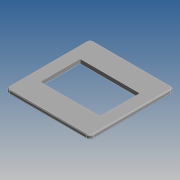
# Autodesk Inventor part: F114DiaReseau
Saved by Autodesk Inventor 2015 SP1 (Build 190203100, 203)
## iProperties
Created: 2017-05-18
Part Number: F114DiaReseau
Material: Générique
Document SubType Name: Modeling
Designer: serge.amoos
Density: 1 g/cm^3
Appearance: Par défaut
Author: serge.amoos
Autodesk Inventor part; units mm, degrees
ref_plane "YZ Plane" through (0, 0, 0) normal (1, 0, 0) x (0, 1, 0)
ref_plane "XZ Plane" through (0, 0, 0) normal (0, 1, 0) x (-1, 0, 0)
ref_plane "XY Plane" through (0, 0, 0) normal (0, 0, 1) x (1, 0, 0)
sketch "Sketch1" plane through (0, 0, 0) normal (0, 0, 1) x (1, 0, 0)
  line L0 (-35.35, 0) -> (35.35, 0) construction
  line L1 (0, -35.35) -> (0, 35.35) construction
  line L2 (-25.25, 25.25) -> (25.25, 25.25)
  line L3 (25.25, 25.25) -> (25.25, -25.25)
  line L4 (25.25, -25.25) -> (-25.25, -25.25)
  line L5 (-25.25, -25.25) -> (-25.25, 25.25)
  line L6 (-18, 12) -> (18, 12)
  line L7 (18, 12) -> (18, -12)
  line L8 (18, -12) -> (-18, -12)
  line L9 (-18, -12) -> (-18, 12)
  point P0 (0, 0)
  point P1 (0, 25.25)
  point P2 (25.25, 0)
  point P3 (0, 12)
  point P4 (18, 0)
  dimension "d0" = 50.5
  dimension "d1" = 50.5
  dimension "d2" = 36
  dimension "d3" = 24
  constraints: 16 end point, 4 midpoint, 4 parallel, 4 point on line, 2 horizontal, 2 perpendicular
  measures "d0" distance of L2.end L3.end
  measures "d1" distance of L2.start L2.end
  measures "d2" distance of L6.start L6.end
  measures "d3" distance of L6.end L7.end
extrude "Extrusion1" add sketch "Sketch1" along normal blind 2.5
fillet "Fillet1" radius 2 4 edges at (-25.25, -25.25, 1.25) (25.25, -25.25, 1.25) (-25.25, 25.25, 1.25) (25.25, 25.25, 1.25)
fillet "Fillet2" radius 0.5 16 edges at (24.6642, -24.6642, 2.5) (25.25, 0, 2.5) (24.6642, 24.6642, 2.5) (0, 25.25, 2.5) (-24.6642, 24.6642, 2.5) (-25.25, 0, 2.5) (-24.6642, -24.6642, 2.5) (0, -25.25, 2.5) (-24.6642, -24.6642, 0) (-25.25, 0, 0) (-24.6642, 24.6642, 0) (0, 25.25, 0) (24.6642, 24.6642, 0) (25.25, 0, 0) (24.6642, -24.6642, 0) (0, -25.25, 0)
equation "\"d1\" = d0"
body "Solid1"
